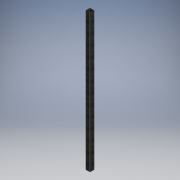
# Autodesk Inventor part: 2350 STEEL PROFILE
Saved by Autodesk Inventor 2018 (Build 220112000, 112)
## iProperties
Created: 2018-10-15
Part Number: 2350 STEEL PROFILE
Material: Acero
Document SubType Name: Modeling
Designer: Toshiba
Density: 7.85 g/cm^3
Appearance: Placa
Author: Toshiba
Autodesk Inventor part; units mm, degrees
ref_plane "YZ Plane" through (0, 0, 0) normal (1, 0, 0) x (0, 1, 0)
ref_plane "XZ Plane" through (0, 0, 0) normal (0, 1, 0) x (-1, 0, 0)
ref_plane "XY Plane" through (0, 0, 0) normal (0, 0, 1) x (1, 0, 0)
sketch "Boceto1" plane through (0, 0, 0) normal (0, 0, 1) x (1, 0, 0)
  line L0 (37.5, -37.5) -> (37.5, 37.5)
  line L1 (37.5, 37.5) -> (-37.5, 37.5)
  line L2 (-37.5, 37.5) -> (-37.5, -37.5)
  line L3 (-37.5, -37.5) -> (37.5, -37.5)
  line L4 (37.5, -37.5) -> (-37.5, 37.5) construction
  line L5 (37.5, 37.5) -> (-37.5, -37.5) construction
  line L6 (-34.5, -34.5) -> (-34.5, 34.5)
  line L7 (-34.5, 34.5) -> (34.5, 34.5)
  line L8 (34.5, 34.5) -> (34.5, -34.5)
  line L9 (34.5, -34.5) -> (-34.5, -34.5)
  point P0 (0, 0)
  dimension "d0" = 75
  dimension "d1" = 75
  dimension "d2" = 3
  constraints: 20 end point, 4 parallel, 2 midpoint, 2 perpendicular, 1 vertical, 3 other
  measures "d0" distance of L0.start L0.end
  measures "d1" distance of L1.end L0.end
  measures "d2" distance between parallel lines of L2 L6
extrude "Extrusión1" add sketch "Boceto1" along normal mid plane 2350
fillet "Empalme1" radius 6 4 edges at (37.5, 37.5, 0) (-37.5, 37.5, 0) (37.5, -37.5, 0) (-37.5, -37.5, 0)
